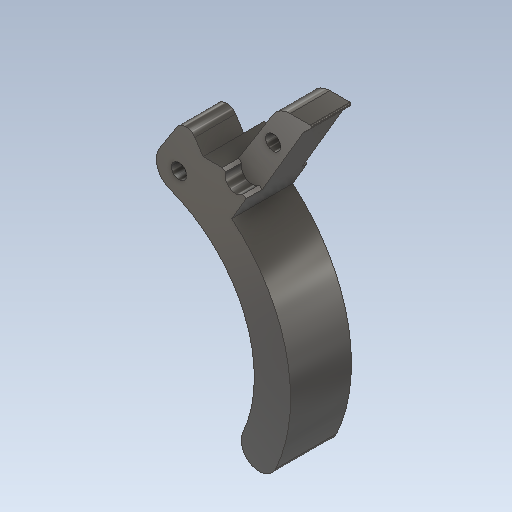
# Autodesk Inventor part: Part43
Saved by Autodesk Inventor 2021 (Build 250183000, 183)
## iProperties
Created: 2020-11-07
Part Number: Part43
Material: Nickel-Copper Alloy 400
Document SubType Name: Modeling
Designer: Lucas Moura
Density: 8.83 g/cm^3
Appearance: Steel - Polished
Author: Lucas Moura
Autodesk Inventor part; units mm, degrees
ref_plane "YZ Plane" through (0, 0, 0) normal (1, 0, 0) x (0, 1, 0)
ref_plane "XZ Plane" through (0, 0, 0) normal (0, 1, 0) x (-1, 0, 0)
ref_plane "XY Plane" through (0, 0, 0) normal (0, 0, 1) x (1, 0, 0)
sketch "Sketch1" plane through (0, 0, 0) normal (0, 0, 1) x (1, 0, 0)
  line L0 (20.6194, 31.3777) -> (22.4899, 31.3777)
  line L1 (22.4899, 31.3777) -> (16.467, 21.1278)
  arc A0 (20.8023, 1.9443) -> (16.467, 21.1278) centre (5.9969, 8.6801) ccw
  line L2 (16.073, 25.8973) -> (18.9256, 30.4411)
  arc A1 (20.6194, 31.3777) -> (18.9256, 30.4411) centre (20.6194, 29.3777) ccw
  line L3 (13.6459, 25.017) -> (15.5204, 25.017)
  line L4 (15.5204, 25.017) -> (16.073, 25.8973)
  arc A2 (17.5545, 3.4219) -> (20.8023, 1.9443) centre (19.1784, 2.6831) ccw
  arc A3 (17.5545, 3.4219) -> (10.3375, 20.6126) centre (5.9969, 8.6801) ccw
  line L5 (9.3399, 23.5753) -> (11.0617, 26.2476)
  line L6 (12.8378, 26.2534) -> (13.6459, 25.017)
  arc A4 (9.3399, 23.5753) -> (10.3375, 20.6126) centre (11.0212, 22.4921) ccw
  arc A5 (12.8378, 26.2534) -> (11.0617, 26.2476) centre (11.9516, 25.6742) ccw
  point P0 (0, 0)
  point P1 (7.8374, 21.2434)
  dimension "d6" = 2
  dimension "d53" = 2
  constraints: 14 end point, 13 point on circle, 6 centre point, 6 tangent, 2 horizontal, 1 coincident, 1 point on line
  measures "d6" radius of A1
  measures "d53" radius of A4
extrude "Extrusion12" add sketch "Sketch1" along normal blind 7
sketch "Sketch14" plane through (0, 0, 7) normal (0, 0, 1) x (1, 0, 0)
  circle A0 centre (11.2711, 22.5911) radius 0.75
  circle A1 centre (18.9401, 28.0713) radius 0.75
  point P0 (0, 0)
  dimension "d56" = 1.5
  dimension "d57" = 1.5
  constraints: 2 centre point
  measures "d56" diameter of A0
  measures "d57" diameter of A1
extrude "Extrusion13" cut sketch "Sketch14" against normal through all
sketch "Sketch15" plane through (0, 0, 0) normal (0, 0, -1) x (-1, 0, 0)
  arc A0 (-12.7572, 23.6392) -> (-10.9318, 20.8046) centre (-11.2711, 22.5911) ccw
  circle A1 centre (-18.9401, 28.0713) radius 0.75 projected
  circle A2 centre (-11.2711, 22.5911) radius 0.75 projected
  line L0 (-22.4899, 31.3777) -> (-20.6194, 31.3777) projected
  line L1 (-16.467, 21.1278) -> (-22.4899, 31.3777) projected
  arc A3 (-16.467, 21.1278) -> (-20.8023, 1.9443) centre (-5.9969, 8.6801) ccw projected
  arc A4 (-20.8023, 1.9443) -> (-17.5545, 3.4219) centre (-19.1784, 2.6831) ccw projected
  arc A5 (-10.3375, 20.6126) -> (-17.5545, 3.4219) centre (-5.9969, 8.6801) ccw projected
  arc A6 (-10.3375, 20.6126) -> (-9.3399, 23.5753) centre (-11.0212, 22.4921) ccw projected
  line L2 (-11.0617, 26.2476) -> (-9.3399, 23.5753) projected
  arc A7 (-11.0617, 26.2476) -> (-12.8378, 26.2534) centre (-11.9516, 25.6742) ccw projected
  line L3 (-13.6459, 25.017) -> (-12.8378, 26.2534) projected
  line L4 (-15.5204, 25.017) -> (-13.6459, 25.017) projected
  line L5 (-18.9256, 30.4411) -> (-15.5204, 25.017) projected
  arc A8 (-18.9256, 30.4411) -> (-20.6194, 31.3777) centre (-20.6194, 29.3777) ccw projected
  line L6 (-10.9318, 20.8046) -> (-10.7125, 20.4694)
  arc A9 (-10.3375, 20.6126) -> (-17.5545, 3.4219) centre (-5.9969, 8.6801) ccw projected
  line L7 (-13.6459, 25.017) -> (-12.7572, 23.6392)
  point P0 (0, 0)
  constraints: 4 end point, 3 point on circle, 1 centre point, 2 other
extrude "Extrusion17" cut sketch "Sketch15" against normal blind 2 contours L7 L3 A7 L2 A6 A5 L6 A0
sketch "Sketch18" plane through (0, 0, 7) normal (0, 0, 1) x (1, 0, 0)
  circle A0 centre (18.9401, 28.0713) radius 0.75 projected
  circle A1 centre (11.2711, 22.5911) radius 0.75 projected
  line L0 (22.4899, 31.3777) -> (20.6194, 31.3777) projected
  arc A2 (20.6194, 31.3777) -> (18.9256, 30.4411) centre (20.6194, 29.3777) ccw projected
  line L1 (18.9256, 30.4411) -> (15.5204, 25.017) projected
  line L2 (15.5204, 25.017) -> (13.6459, 25.017) projected
  line L3 (13.6459, 25.017) -> (12.8378, 26.2534) projected
  arc A3 (12.8378, 26.2534) -> (11.0617, 26.2476) centre (11.9516, 25.6742) ccw projected
  line L4 (11.0617, 26.2476) -> (9.3399, 23.5753) projected
  arc A4 (9.3399, 23.5753) -> (10.3375, 20.6126) centre (11.0212, 22.4921) ccw projected
  arc A5 (17.5545, 3.4219) -> (10.3375, 20.6126) centre (5.9969, 8.6801) ccw projected
  arc A6 (17.5545, 3.4219) -> (20.8023, 1.9443) centre (19.1784, 2.6831) ccw projected
  arc A7 (20.8023, 1.9443) -> (16.467, 21.1278) centre (5.9969, 8.6801) ccw projected
  line L5 (16.467, 21.1278) -> (22.4899, 31.3777) projected
  line L6 (16.467, 21.1278) -> (22.4899, 31.3777) projected
  line L7 (15.5204, 25.017) -> (15.8591, 24.8043)
  line L8 (17.8813, 23.5348) -> (17.5365, 23.7374)
  arc A8 (15.8591, 24.8043) -> (17.5365, 23.7374) centre (16.8393, 24.4933) ccw
  point P0 (0, 0)
  dimension "d75" = 0.4
  dimension "d76" = 0.4
  constraints: 4 end point, 2 perpendicular, 2 point on circle, 1 centre point, 1 point on line
  measures "d75" distance of L1.end L7.end
  measures "d76" distance of L8.start L8.end
extrude "Extrusion18" cut sketch "Sketch18" against normal blind 2.605 contours L5 L8 A8 L7 L1 A2 L0
sketch "Sketch19" plane through (12.7572, 23.6392, 0) normal (-0.8403389, 0.5420613, 0) x (0, 0, 1)
  line L0 (0, 0) -> (0, 1.6395) projected
  line L1 (0, 0) -> (2, 0) projected
  line L2 (2, 0) -> (2, 1.6395) projected
  line L3 (0, 1.6395) -> (2, 1.6395) projected
  circle A0 centre (1, 0.8198) radius 0.25
  line L4 (0, 0) -> (2, 0) projected
  line L5 (2, 1.6395) -> (0, 0)
  line L6 (0, 0) -> (0, 1.6395)
  line L7 (2, 0) -> (0, 1.6395)
  point P0 (0, -26.7801)
  dimension "d79" = 0.5
  constraints: 6 end point, 1 centre point, 1 perpendicular
  measures "d79" diameter of A0
extrude "Extrusion19" cut sketch "Sketch19" against normal blind 1 contours L5 L7 A0 | A0 L7 L5 | A0 L5 L7 | L7 L5 A0
sketch "Sketch20" plane through (22.4899, 31.3777, 0) normal (0, 0, -1) x (-1, 0, 0)
  line L0 (11.7774, -10.9083) -> (11.5581, -10.5731) projected
  arc A0 (9.7327, -7.7385) -> (11.5581, -10.5731) centre (11.2188, -8.7866) ccw projected
  line L1 (9.7327, -7.7385) -> (8.844, -6.3607) projected
  line L2 (6.9695, -6.3607) -> (8.844, -6.3607) projected
  line L3 (3.5643, -0.9366) -> (6.9695, -6.3607) projected
  arc A1 (3.5643, -0.9366) -> (1.8705, 0) centre (1.8705, -2) ccw projected
  line L4 (0, 0) -> (1.8705, 0) projected
  line L5 (6.0229, -10.2499) -> (0, 0) projected
  arc A2 (6.0229, -10.2499) -> (1.6876, -29.4334) centre (16.493, -22.6976) ccw projected
  arc A3 (1.6876, -29.4334) -> (4.9355, -27.9558) centre (3.3115, -28.6946) ccw projected
  arc A4 (11.7774, -10.9083) -> (4.9355, -27.9558) centre (16.493, -22.6976) ccw projected
  circle A5 centre (3.5498, -3.3064) radius 0.75 projected
  line L6 (6.6308, -6.5734) -> (6.9695, -6.3607) projected
  arc A6 (4.9534, -7.6403) -> (6.6308, -6.5734) centre (5.6506, -6.8844) ccw projected
  line L7 (4.6086, -7.8429) -> (4.9534, -7.6403) projected
  point P0 (22.4899, -31.3777)
extrude "Extrusion20" cut sketch "Sketch20" against normal blind 0.475 contours L6 A6 L7 L5 L4 A1 L3
sketch "Sketch22" plane through (20.6194, 31.3777, 4.395) normal (0, 0, 1) x (1, 0, 0)
  circle A0 centre (-1.6793, -3.3064) radius 0.75 projected
  line L0 (0, 0) -> (1.8705, 0) projected
  arc A1 (0, 0) -> (-1.6939, -0.9366) centre (0, -2) ccw projected
  line L1 (-5.0991, -6.3607) -> (-1.6939, -0.9366) projected
  line L2 (-4.7603, -6.5734) -> (-5.0991, -6.3607) projected
  arc A2 (-4.7603, -6.5734) -> (-3.083, -7.6403) centre (-3.7801, -6.8844) ccw projected
  line L3 (-2.7381, -7.8429) -> (-3.083, -7.6403) projected
  line L4 (1.8705, 0) -> (-2.7381, -7.8429) projected
  line L5 (0, 0) -> (2.0726, 0)
  line L6 (2.0726, 0) -> (2.0726, -0.23)
  arc A3 (2.0726, -0.23) -> (0.5611, -2.2282) centre (5.2352, -4.1929) ccw
  point P0 (-20.6194, -31.3777)
  point P1 (1.2441, -1.066)
  dimension "d99" = 0.23
  constraints: 4 end point, 2 point on circle, 1 centre point, 1 horizontal, 1 point on line, 1 vertical
  measures "d99" distance of L5.end L6.end
extrude "Extrusion22" add sketch "Sketch22" against normal up to surface (3.92 mm away) contours L5 L6 A3 L4
fillet "Fillet8" radius 0.1 2 edges at (22.6921, 31.1477, 2.435) (22.6921, 31.3777, 2.435)
sketch "Sketch23" plane through (0, 0, 7) normal (0, 0, 1) x (1, 0, 0)
  line L0 (15.8591, 24.8043) -> (15.5204, 25.017) projected
  line L1 (15.5204, 25.017) -> (13.6459, 25.017) projected
  line L2 (13.6459, 25.017) -> (12.8378, 26.2534) projected
  arc A0 (12.8378, 26.2534) -> (11.0617, 26.2476) centre (11.9516, 25.6742) ccw projected
  line L3 (11.0617, 26.2476) -> (9.3399, 23.5753) projected
  arc A1 (9.3399, 23.5753) -> (10.3375, 20.6126) centre (11.0212, 22.4921) ccw projected
  arc A2 (17.5545, 3.4219) -> (10.3375, 20.6126) centre (5.9969, 8.6801) ccw projected
  arc A3 (17.5545, 3.4219) -> (20.8023, 1.9443) centre (19.1784, 2.6831) ccw projected
  arc A4 (20.8023, 1.9443) -> (16.467, 21.1278) centre (5.9969, 8.6801) ccw projected
  line L4 (16.467, 21.1278) -> (17.8813, 23.5348) projected
  line L5 (17.8813, 23.5348) -> (17.5365, 23.7374) projected
  arc A5 (15.8591, 24.8043) -> (17.5365, 23.7374) centre (16.8393, 24.4933) ccw projected
  circle A6 centre (11.2711, 22.5911) radius 0.75 projected
  point P0 (0, 0)
extrude "Extrusion23" cut sketch "Sketch23" against normal blind 1
body "Solid1"
body "Solid3"
